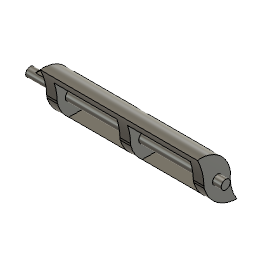
BeaterBar_v2 (Autodesk Fusion 360 design; units mm, degrees)
part number: 2026-06-15-17-33-51-553
Autodesk Fusion 360 part; units mm, degrees
sketch "Sketch1" plane through (0, 0, 0) normal (1, 0, 0) x (0, 0, -1)
  circle A0 centre (0, 0) radius 3.9
  arc A1 (10.0577, 0) -> (-15, 20) centre (-12.7457, -2.8729) ccw
  arc A2 (-10.0577, 0) -> (-15, 20) centre (-52.9962, 0) ccw
  arc A3 (-10.0577, 0) -> (15, -20) centre (15.3991, 6.1973) ccw
  arc A4 (10.0577, 0) -> (15, -20) centre (39.3048, -3.3833) ccw
  dimension "d1" = 7.8
  constraint coincident A0.centre origin
  measures "d1" diameter of A0
extrude "Extrude1" add sketch "Sketch1" along normal blind 119 contours A0 | A1 A2 A3 A4
sketch "Sketch2" plane through (0, 0, 0) normal (-1, 0, 0) x (0, 0, 1)
  arc A0 (-15, -20) -> (10.0577, 0) centre (-15.3991, 6.1973) ccw
  arc A1 (15, 20) -> (10.0577, 0) centre (52.9962, 0) ccw
  arc A2 (15, 20) -> (-10.0577, 0) centre (12.7457, -2.8729) ccw
  arc A3 (-15, -20) -> (-10.0577, 0) centre (-39.3048, -3.3833) ccw
  line L0 (18, 14) -> (-18, 14)
  line L1 (-18, 14) -> (-18, -14)
  line L2 (-18, -14) -> (18, -14)
  line L3 (18, -14) -> (18, 14)
  line L4 (18, 14) -> (-18, -14) construction
  line L5 (-18, 14) -> (18, -14) construction
  dimension "d5" = 28
  dimension "d6" = 36
  constraint horizontal L0
  constraint perpendicular L0 L1
  constraint parallel L0 L2
  constraint parallel L1 L3
  constraint coincident L4 origin
  constraint coincident L5 origin
  measures "d5" distance of L0.end L1.end
  measures "d6" distance of L0.start L0.end
extrude "Extrude2" cut sketch "Sketch2" against normal blind 47.5 from surface at -8 contours A0 A1 A2 A3 L0 L2
sketch "Sketch3" plane through (0, 0, 0) normal (-1, 0, 0) x (0, 0, 1)
  arc A0 (-15, -20) -> (10.0577, 0) centre (-15.3991, 6.1973) ccw
  arc A1 (15, 20) -> (10.0577, 0) centre (52.9962, 0) ccw
  arc A2 (15, 20) -> (-10.0577, 0) centre (12.7457, -2.8729) ccw
  arc A3 (-15, -20) -> (-10.0577, 0) centre (-39.3048, -3.3833) ccw
  line L0 (-18, 14) -> (18, 14)
  line L1 (18, 14) -> (18, -14)
  line L2 (18, -14) -> (-18, -14)
  line L3 (-18, -14) -> (-18, 14)
  line L4 (-18, 14) -> (18, -14) construction
  line L5 (18, 14) -> (-18, -14) construction
  constraint horizontal L0
  constraint perpendicular L0 L1
  constraint parallel L0 L2
  constraint parallel L1 L3
  constraint coincident L4 origin
  constraint coincident L5 origin
extrude "Extrude3" cut sketch "Sketch3" against normal blind 47.5 from surface at -63.5 contours A0 A1 A2 A3 L0 L2
sketch "Sketch4" plane through (0, 0, 0) normal (-1, 0, 0) x (0, 0, 1)
  arc A0 (-15, -20) -> (10.0577, 0) centre (-15.3991, 6.1973) ccw
  arc A1 (15, 20) -> (10.0577, 0) centre (52.9962, 0) ccw
  arc A2 (15, 20) -> (-10.0577, 0) centre (12.7457, -2.8729) ccw
  arc A3 (-15, -20) -> (-10.0577, 0) centre (-39.3048, -3.3833) ccw
  circle A4 centre (0, 0) radius 3.9
  dimension "d13" = 7.8
  constraint coincident A4.centre origin
  measures "d13" diameter of A4
extrude "Extrude4" add sketch "Sketch4" along normal blind 23 and the other way blind 126 contours A4
sketch "Sketch5" plane through (-23, 0, 0) normal (-1, 0, 0) x (0, 0, 1)
  circle A0 centre (0, 0) radius 3.9
  line L0 (-2.4987, 2.9944) -> (2.4987, 2.9944)
  line L1 (-2.4987, 2.9944) -> (-2.4987, -2.9944)
  constraint coincident A0 L0.start
  constraint coincident A0 L0.end
  constraint horizontal L0
  constraint coincident A0 L1.end
  constraint perpendicular L0 L1
extrude "Extrude5" cut sketch "Sketch5" against normal blind 23 contours A0 L0 | A0 L1
sketch "Sketch6" plane through (126, 0, 0) normal (1, 0, 0) x (0, 0, -1)
  circle A0 centre (0, 0) radius 3.9
  line L0 (-3.4996, 1.7212) -> (-3.4996, -1.7212)
  line L1 (-1.7089, -3.5056) -> (1.7089, -3.5056)
  line L2 (3.4996, -1.7212) -> (3.4996, 1.7212)
  line L3 (-1.5, 3.6) -> (1.5, 3.6)
  constraint coincident A0 L0.start
  constraint coincident A0 L0.end
  constraint coincident A0 L1.start
  constraint coincident A0 L1.end
  constraint perpendicular L0 L1
  constraint coincident A0 L2.start
  constraint coincident A0 L2.end
  constraint perpendicular L1 L2
  constraint coincident A0 L3.start
  constraint coincident A0 L3.end
  constraint horizontal L3
extrude "Extrude6" cut sketch "Sketch6" against normal blind 7 contours A0 L2 | A0 L3 | A0 L1 | A0 L0
fillet "Fillet1" radius 7 3 edges at (59.5, 0, 10.0577) (4, 0, 10.0577) (115, 0, 10.0577)
fillet "Fillet2" radius 7 3 edges at (59.5, 0, -10.0577) (115, 0, -10.0577) (4, 0, -10.0577)
extrude "Extrude7" cut 1 faces at (126, -1.1371, 0.5) along direction (-1, 0, 0) blind 0.5
extrude "Extrude8" cut 1 faces at (-23, 0.5875, 0.4005) along direction (1, 0, 0) blind 0.5
extrude "Extrude9" cut 1 faces at (-22.5, 0.5875, 0.4005) along direction (1, 0, 0) blind 22.5
sketch "Sketch7" plane through (0, 0, 0) normal (-1, 0, 0) x (0, 0, 1)
  arc A0 (-9.904, 1.0312) -> (-9.9782, -0.7774) centre (-3.0057, -0.1579) ccw
  arc A1 (-15, -20) -> (-9.9782, -0.7774) centre (-39.3048, -3.3833) ccw
  arc A2 (-15, -20) -> (9.7987, -0.9811) centre (-15.3991, 6.1973) ccw
  arc A3 (9.7987, -0.9811) -> (10.0653, 0.8055) centre (3.0665, 0.9368) ccw
  arc A4 (15, 20) -> (10.0653, 0.8055) centre (52.9962, 0) ccw
  arc A5 (15, 20) -> (-9.904, 1.0312) centre (12.7457, -2.8729) ccw
  circle A6 centre (0, 0) radius 3.5
  dimension "d32" = 7
  constraint coincident A6.centre origin
  measures "d32" diameter of A6
extrude "Extrude10" add sketch "Sketch7" along normal blind 22.5 contours A6
sketch "Sketch8" plane through (-22.5, 0, 0) normal (-1, 0, 0) x (0, 0, 1)
  circle A0 centre (0, 0) radius 3.5
  line L0 (-1.8028, 3) -> (1.8028, 3)
  line L1 (-3, 1.8028) -> (-3, -1.8028)
  dimension "d35" = 3
  dimension "d36" = 3
  constraint coincident A0 L0.start
  constraint coincident A0 L0.end
  constraint horizontal L0
  constraint coincident A0 L1.start
  constraint coincident A0 L1.end
  constraint perpendicular L0 L1
  measures "d35" distance of A0.centre L0
  measures "d36" distance of A0.centre L1
extrude "Extrude11" cut sketch "Sketch8" against normal blind 16.5 from surface at -6 contours A0 L0 | A0 L1
extrude "Extrude12" cut 1 faces at (125.5, -1.1371, 0.5) along direction (-1, 0, 0) blind 6.5
sketch "Sketch9" plane through (119, 0, 0) normal (1, 0, 0) x (0, 0, -1)
  arc A0 (9.9782, -0.7774) -> (9.904, 1.0312) centre (3.0057, -0.1579) ccw
  arc A1 (9.904, 1.0312) -> (-15, 20) centre (-12.7457, -2.8729) ccw
  arc A2 (-10.0653, 0.8055) -> (-15, 20) centre (-52.9962, 0) ccw
  arc A3 (-10.0653, 0.8055) -> (-9.7987, -0.9811) centre (-3.0665, 0.9368) ccw
  arc A4 (-9.7987, -0.9811) -> (15, -20) centre (15.3991, 6.1973) ccw
  arc A5 (9.9782, -0.7774) -> (15, -20) centre (39.3048, -3.3833) ccw
  circle A6 centre (0, 0) radius 3.5
  dimension "d42" = 7
  constraint coincident A6.centre origin
  measures "d42" diameter of A6
extrude "Extrude13" add sketch "Sketch9" along normal blind 6.5 contours A6
